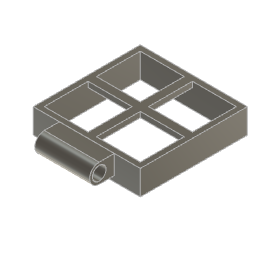
Left EWI with Bumps v5 (Autodesk Fusion 360 archive; units mm, degrees)
design "UFC Warning Cover"
Autodesk Fusion 360 part; units mm, degrees
sketch "Sketch1" plane through (0, 0, 0) normal (0, 0, 1) x (1, 0, 0)
  line L0 (8.75, -8.75) -> (-8.75, -8.75)
  line L1 (-8.75, -8.75) -> (-8.75, 8.75)
  line L2 (-8.75, 8.75) -> (8.75, 8.75)
  line L3 (8.75, 8.75) -> (8.75, -8.75)
  line L4 (8.75, -8.75) -> (-8.75, 8.75) construction
  line L5 (-8.75, -8.75) -> (8.75, 8.75) construction
  line L6 (9.75, -9.75) -> (-9.75, -9.75)
  line L7 (-9.75, -9.75) -> (-9.75, 9.75)
  line L8 (-9.75, 9.75) -> (9.75, 9.75)
  line L9 (9.75, 9.75) -> (9.75, -9.75)
  line L10 (9.75, -9.75) -> (-9.75, 9.75) construction
  line L11 (-9.75, -9.75) -> (9.75, 9.75) construction
  dimension "d1" = 17.5
  dimension "d2" = 17.5
  dimension "d3" = 19.5
  dimension "d4" = 19.5
  constraint horizontal L0
  constraint perpendicular L0 L1
  constraint parallel L0 L2
  constraint parallel L1 L3
  constraint coincident L4 origin
  constraint coincident L5 origin
  constraint horizontal L6
  constraint perpendicular L6 L7
  constraint parallel L6 L8
  constraint parallel L7 L9
  constraint coincident L10 origin
  constraint coincident L11 origin
  measures "d1" distance of L1.end L2.end
  measures "d2" distance of L0.end L1.end
  measures "d3" distance of L7.end L8.end
  measures "d4" distance of L6.end L7.end
extrude "Extrude1" add sketch "Sketch1" along normal blind 3.5
sketch "Sketch2" plane through (0, 0, 3.5) normal (0, 0, 1) x (-1, 0, 0)
  line L0 (8.75, -8.75) -> (-8.75, -8.75)
  line L1 (-8.75, -8.75) -> (-8.75, 8.75)
  line L2 (-8.75, 8.75) -> (8.75, 8.75)
  line L3 (8.75, 8.75) -> (8.75, -8.75)
  line L4 (-9.75, -9.75) -> (9.75, -9.75)
  line L5 (9.75, -9.75) -> (9.75, 9.75)
  line L6 (9.75, 9.75) -> (-9.75, 9.75)
  line L7 (-9.75, 9.75) -> (-9.75, -9.75)
  line L8 (0.75, -9.75) -> (-0.75, -9.75)
  line L9 (-0.75, -9.75) -> (-0.75, 9.75)
  line L10 (-0.75, 9.75) -> (0.75, 9.75)
  line L11 (0.75, 9.75) -> (0.75, -9.75)
  line L12 (0.75, -9.75) -> (-0.75, 9.75) construction
  line L13 (-0.75, -9.75) -> (0.75, 9.75) construction
  line L14 (9.75, -0.75) -> (-9.75, -0.75)
  line L15 (-9.75, -0.75) -> (-9.75, 0.75)
  line L16 (-9.75, 0.75) -> (9.75, 0.75)
  line L17 (9.75, 0.75) -> (9.75, -0.75)
  line L18 (9.75, -0.75) -> (-9.75, 0.75) construction
  line L19 (-9.75, -0.75) -> (9.75, 0.75) construction
  dimension "d7" = 1.5
  dimension "d8" = 1.5
  constraint horizontal L8
  constraint perpendicular L8 L9
  constraint parallel L8 L10
  constraint parallel L9 L11
  constraint coincident L12 origin
  constraint coincident L13 origin
  constraint horizontal L14
  constraint perpendicular L14 L15
  constraint parallel L14 L16
  constraint parallel L15 L17
  constraint coincident L18 origin
  constraint coincident L19 origin
  measures "d7" distance of L9.end L10.end
  measures "d8" distance of L14.end L15.end
extrude "Extrude2" add sketch "Sketch2" along normal blind 1 contours L0 L3 L4 L5 L11 L14 | L0 L4 L8 L9 L11 | L0 L9 L11 L14 | L3 L11 L14 L16 | L3 L5 L14 L16 L17 | L0 L1 L4 L7 L9 L14 | L9 L11 L14 L16 | L2 L3 L5 L6 L11 L16 | L1 L9 L14 L16 | L2 L9 L11 L16 | L1 L7 L14 L15 L16 | L2 L6 L9 L10 L11 | L1 L2 L6 L7 L9 L16
ref_plane "WorkPlane1" through (0, 0, 2.25) normal (1, 0, 0) x (0, 1, 0)
sketch "Sketch3" plane through (0, 0, 2.25) normal (1, 0, 0) x (0, 1, 0)
  line L0 (-9.7484, 2.2378) -> (-12.4984, 2.2378)
  line L1 (-12.4984, 2.2378) -> (-12.4984, -0.5122)
  line L2 (-12.4984, -0.5122) -> (-9.7484, -0.5122)
  line L3 (-9.7484, -0.5122) -> (-9.7484, 2.2378)
  circle A0 centre (-12.4831, 0.4878) radius 1.75
  circle A1 centre (-12.4831, 0.4878) radius 1.2499
  line L4 (-9.7484, -0.5122) -> (-12.4754, -0.5122)
  line L5 (-12.4754, -0.5122) -> (-12.4754, -1.2622)
  line L6 (-12.4754, -1.2622) -> (-9.7484, -1.2622)
  line L7 (-9.7484, -1.2622) -> (-9.7484, -0.5122)
  dimension "d12" = 2.75
  dimension "d13" = 2.75
  dimension "d14" = 3.5
  dimension "d15" = 2.4999
  constraint horizontal L0
  constraint vertical L1
  constraint horizontal L2
  constraint vertical L3
  constraint coincident L0.end A0
  constraint concentric A0 A1
  constraint horizontal L4
  constraint vertical L5
  constraint horizontal L6
  constraint vertical L7
  constraint coincident A0 L5.end
  measures "d12" distance of L0.start L0.end
  measures "d13" distance of L0.start L2.end
  measures "d14" diameter of A0
  measures "d15" diameter of A1
extrude "Extrude3" add sketch "Sketch3" along normal blind 5 contours L1 L2 A0 A1 L4 | L1 A0 A1 L5 | L0 L2 L3 A0 L4 | L2 A0 L4 L6 L7 | L2 A0 A1 L4 L5
extrude "Extrude4" add sketch "Sketch3" against normal blind 5 contours L1 L2 A0 A1 L4 | L1 A0 A1 L5 | L0 L2 L3 A0 L4 | L2 A0 L4 L6 L7 | L2 A0 A1 L4 L5
